# Autodesk Inventor part: TXB0108PWR
Saved by Autodesk Inventor 2013 (Build 170138000, 138)
## iProperties
Created: 2013-01-27
Part Number: TXB0108PWR
Material: Generic
Document SubType Name: Modeling
Designer: davidgitz
Density: 1 g/cm^3
Author: davidgitz
Autodesk Inventor part; units mm, degrees
ref_plane "YZ Plane" through (0, 0, 0) normal (1, 0, 0) x (0, 1, 0)
ref_plane "XZ Plane" through (0, 0, 0) normal (0, 1, 0) x (-1, 0, 0)
ref_plane "XY Plane" through (0, 0, 0) normal (0, 0, 1) x (1, 0, 0)
sketch "R-PDSO-G20, TXB0108PWR_35" plane through (0, 0, 0) normal (0, 0, 1) x (1, 0, 0)
  line L0 (-3.125, 2.1001) -> (3.125, 2.1001)
  line L1 (3.125, 2.1001) -> (3.125, -2.1001)
  line L2 (3.125, -2.1001) -> (-3.125, -2.1001)
  line L3 (-3.125, -2.1001) -> (-3.125, -0.3749)
  line L4 (-3.125, -0.3749) -> (-2.7501, -0.3749)
  line L5 (-2.7501, -0.3749) -> (-2.7501, 0.3749)
  line L6 (-2.7501, 0.3749) -> (-3.125, 0.3749)
  line L7 (-3.125, 0.3749) -> (-3.125, 2.1001)
  constraints: 16 end point
extrude "Extrusion1" add sketch "R-PDSO-G20, TXB0108PWR_35" along normal blind 6.35
body "Solid1"
